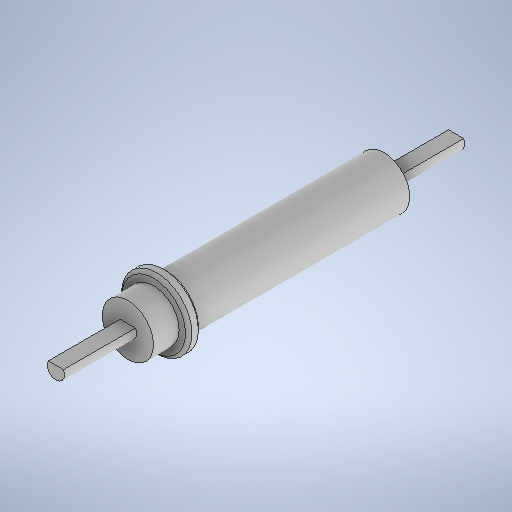
# Autodesk Inventor part: axle-skibidi
Saved by Autodesk Inventor 2025.1 (Build 291241020, 241B)
## iProperties
Created: 2024-08-26
Part Number: axle-skibidi
Material: Generic
Document SubType Name: Modeling
Designer: limfe
Density: 1 g/cm^3
Appearance: Default
Author: limfe
Autodesk Inventor part; units mm, degrees
ref_plane "YZ Plane" through (0, 0, 0) normal (1, 0, 0) x (0, 1, 0)
ref_plane "XZ Plane" through (0, 0, 0) normal (0, 1, 0) x (-1, 0, 0)
sketch "Sketch1" plane through (0, 0, 0) normal (0, 1, 0) x (-1, 0, 0)
  circle A0 centre (0, 0) radius 4
  dimension "d0" = 8
  constraints: 2 coincident, 1 centre point
  measures "d0" diameter of A0
extrude "Extrusion1" add sketch "Sketch1" along normal blind 36
sketch "Sketch3" plane through (0, 0, 0) normal (0, -1, 0) x (1, 0, 0)
  line L0 (-1.1832, 0.85) -> (1.1832, 0.85)
  arc A0 (-1.1832, 0.85) -> (1.1832, 0.85) centre (0, 0.2) ccw
  point P0 (0, 0)
  point P1 (0, 0)
  point P2 (0, 0.85)
  dimension "d16" = 1.35
  dimension "d17" = 0.2
  dimension "d39" = 2
  constraints: 2 coincident, 2 end point, 2 point on circle, 1 centre point, 1 horizontal, 1 midpoint, 1 vertical alignment
  measures "d16" radius of A0
  measures "d17" distance of point (0, 0) A0.centre
extrude "Extrusion3" add sketch "Sketch3" along normal blind 15.25
sketch "Sketch5" plane through (0, 0, 0) normal (0, -1, 0) x (1, 0, 0)
  circle A0 centre (0, 0) radius 5.5
  dimension "d29" = 11
  constraints: 1 centre point, 1 coincident
  measures "d29" diameter of A0
extrude "Extrusion5" add sketch "Sketch5" against normal blind 2
chamfer "Chamfer3" distance 0.5 angle 45 2 edges at (-5.5, 0, 0) (-5.5, 2, 0)
sketch "Sketch6" plane through (0, 0, 0) normal (0, -1, 0) x (1, 0, 0)
  circle A0 centre (0, 0) radius 5 projected
  line L0 (-7.7, 0) -> (7.7, 0) projected
  line L1 (0, -7.7) -> (0, 7.7) projected
  circle A1 centre (0, 0) radius 4
  dimension "d35" = 8
  constraints: 1 centre point, 1 coincident
  measures "d35" diameter of A1
extrude "Extrusion6" add sketch "Sketch6" along normal blind 4 contours A1 L1 L0 | L0 L1 A1 | L1 L0 A1 | A1 L0 L1
ref_plane "Work Plane1" through (0, 16, 0) normal (0, 1, 0) x (1, 0, 0)
mirror "Mirror1" about plane through (0, 16, 0) normal (0, 1, 0) of "Extrusion3"
body "Solid1"
